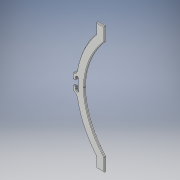
# Autodesk Inventor part: Baseplate_aussen
Saved by Autodesk Inventor 2018 (Build 220112000, 112)
## iProperties
Created: 2020-01-15
Part Number: Baseplate_aussen
Material: Generisch
Document SubType Name: Modeling
Designer: maxse
Density: 1 g/cm^3
Appearance: Vorgabe
Author: maxse
Autodesk Inventor part; units mm, degrees
ref_plane "YZ Plane" through (0, 0, 0) normal (1, 0, 0) x (0, 1, 0)
ref_plane "XZ Plane" through (0, 0, 0) normal (0, 1, 0) x (-1, 0, 0)
ref_plane "XY Plane" through (0, 0, 0) normal (0, 0, 1) x (1, 0, 0)
sketch "Skizze1" plane through (0, 0, 0) normal (0, 1, 0) x (-1, 0, 0)
  arc A0 (39, 0) -> (0, 95) centre (-110.879, -6.024) ccw
  line L0 (0, 95) -> (0, 120)
  line L1 (0, 120) -> (15, 120)
  line L2 (15, 120) -> (15, 100.6336)
  arc A1 (54, 0) -> (15, 100.6336) centre (-110.879, -6.024) ccw
  line L3 (39, 0) -> (54, 0)
  line L4 (0, 0) -> (39, 0)
  line L5 (59, 0) -> (59, 15)
  line L6 (59, 15) -> (52.765, 15)
  line L7 (59, 0) -> (54, 0)
  dimension "d0" = 25
  dimension "d2" = 15
  dimension "d4" = 54
  dimension "d5" = 0
  dimension "d6" = 120
  dimension "d7" = 150
  dimension "d9" = 5
  dimension "d10" = 15
  dimension "d11" = 15
  constraints: 16 end point, 6 point on circle, 3 perpendicular, 2 centre point, 2 horizontal, 2 vertical, 1 collinear, 1 concentric
  measures "d0" distance of L0.start L0.end
  measures "d2" distance of L0.end L1.end
  measures "d4" distance of L3.end L4.start
  measures "d5" distance from line of L4.start L0
  measures "d6" distance from line of L4.start L1
  measures "d7" radius of A0
  measures "d9" distance of L3.end L5.start
  measures "d10" distance of L3.end L3.start
  measures "d11" distance of L5.start L5.end
extrude "Extrusion1" add sketch "Skizze1" along normal blind 4
mirror "Spiegeln1" about plane through (-54, 0, 0) normal (0, 0, -1) of "Extrusion1"
sketch "Skizze2" plane through (0, 0, 0) normal (0, -1, 0) x (1, 0, 0)
  line L0 (-59, 15) -> (-59, -15) projected
  line L1 (-59, -5) -> (-54, -5)
  line L2 (-54, -5) -> (-54, -9.5)
  line L3 (-59, 5) -> (-54, 5)
  line L4 (-54, 5) -> (-54, 9.5)
  line L5 (-49, -9.5) -> (-49, 9.5)
  arc A0 (-49, 9.5) -> (-54, 9.5) centre (-51.5, 9.5) ccw
  arc A1 (-54, -9.5) -> (-49, -9.5) centre (-51.5, -9.5) ccw
  point P0 (0, 0)
  dimension "d15" = 10
  dimension "d16" = 5
  dimension "d17" = 10
  dimension "d18" = 5
  dimension "d19" = 5
  dimension "d20" = 24
  dimension "d21" = 4.5
  constraints: 10 end point, 4 point on circle, 4 tangent, 2 centre point, 2 horizontal, 2 point on line, 2 vertical, 1 perpendicular
  measures "d15" distance between parallel lines of L5 L0
  measures "d16" distance between parallel lines of L5 L2
  measures "d17" distance between parallel lines of L3 L1
  measures "d18" distance of L3.start L3.end
  measures "d19" distance from line of point (0, 0) L3
  measures "d21" distance from line of L1 A1.centre
extrude "Extrusion2" cut sketch "Skizze2" against normal blind 4
fillet "Rundung1" radius 10 3 edges at (-52.765, 2, -15) (-52.765, 2, 15) (-39, 2, 0)
fillet "Rundung2" radius 1 46 edges at (-7.5, 4, -120) (0, 4, -107.5) (-15, 4, -110.3168) (-7.5, 0, -120) (0, 0, -107.5) (-15, 0, -110.3168) (-54.0935, 4, -17.8718) (-38.4134, 4, -64.2123) (-54.0935, 0, -17.8718) (-38.4134, 0, -64.2123) (-38.9913, 4, 0) (-27.8012, 4, 51.1406) (-27.8012, 4, -51.1406) (-38.9913, 0, 0) (-27.8012, 0, 51.1406) (-27.8012, 0, -51.1406) (-54.0935, 4, 17.8718) (-38.4134, 4, 64.2123) (-54.0935, 0, 17.8718) (-38.4134, 0, 64.2123) (-59, 4, 10) (-59, 0, 10) (-59, 0, -10) (-59, 4, -10) (-59, 2, -5) (-59, 2, 5) (-54, 2, 5) (-54, 2, -5) (-56.5, 4, -5) (-56.5, 4, 5) (-51.5, 4, 12) (-54, 4, 7.25) (-51.5, 4, -12) (-54, 4, -7.25) (-49, 4, 0) (-51.5, 0, -12) (-54, 0, -7.25) (-51.5, 0, 12) (-54, 0, 7.25) (-49, 0, 0) (-15, 4, 110.3168) (-15, 0, 110.3168) (-7.5, 4, 120) (-7.5, 0, 120) (0, 0, 107.5) (0, 4, 107.5)
sketch "Skizze3" plane through (0, 4, 0) normal (0, 1, 0) x (1, 0, 0)
  line L0 (-45.0909, 10.6088) -> (-45.0909, 11.0512)
  line L1 (-45.0909, 11.0512) -> (-44.8243, 11.0512)
  spline S0 degree 2 poles (-44.8243, 11.0512) (-44.9094, 11.1533) (-45.0228, 11.3036) (-45.0711, 11.4058) knots 0 0 0 1 2 2 2
  spline S1 degree 2 poles (-45.0711, 11.4058) (-45.1164, 11.4994) (-45.1647, 11.7007) (-45.1647, 11.834) knots 0 0 0 1 2 2 2
  spline S2 degree 2 poles (-45.1647, 11.834) (-45.1647, 12.0496) (-44.986, 12.4126) (-44.813, 12.5403) knots 0 0 0 1 2 2 2
  spline S3 degree 2 poles (-44.813, 12.5403) (-44.6399, 12.6679) (-44.1294, 12.8097) (-43.7976, 12.8097) knots 0 0 0 1 2 2 2
  spline S4 degree 2 poles (-43.7976, 12.8097) (-43.4515, 12.8097) (-42.9467, 12.631) (-42.7566, 12.475) knots 0 0 0 1 2 2 2
  spline S5 degree 2 poles (-42.7566, 12.475) (-42.5865, 12.3304) (-42.3908, 11.9248) (-42.3908, 11.7007) knots 0 0 0 1 2 2 2
  spline S6 degree 2 poles (-42.3908, 11.7007) (-42.3908, 11.505) (-42.4787, 11.2129) (-42.5694, 11.0512) knots 0 0 0 1 2 2 2
  line L2 (-42.5694, 11.0512) -> (-41.4349, 11.0512)
  line L3 (-41.4349, 11.0512) -> (-41.4349, 10.6088)
  line L4 (-41.4349, 10.6088) -> (-45.0909, 10.6088)
  line L5 (-44.4528, 11.0512) -> (-42.9353, 11.0512)
  spline S7 degree 2 poles (-42.9353, 11.0512) (-42.8559, 11.2157) (-42.7964, 11.4767) (-42.7964, 11.627) knots 0 0 0 1 2 2 2
  spline S8 degree 2 poles (-42.7964, 11.627) (-42.7964, 11.9673) (-43.3069, 12.3531) (-43.7891, 12.3531) knots 0 0 0 1 2 2 2
  spline S9 degree 2 poles (-43.7891, 12.3531) (-44.2542, 12.3531) (-44.7449, 12.0581) (-44.7449, 11.7319) knots 0 0 0 1 2 2 2
  spline S10 degree 2 poles (-44.7449, 11.7319) (-44.7449, 11.5589) (-44.5861, 11.2072) (-44.4528, 11.0512) knots 0 0 0 1 2 2 2
  spline S11 degree 2 poles (-45.1505, 8.8276) (-45.1505, 9.4572) (-44.4442, 10.1493) (-43.7919, 10.1493) knots 0 0 0 1 2 2 2
  spline S12 degree 2 poles (-43.7919, 10.1493) (-43.1509, 10.1493) (-42.3908, 9.4771) (-42.3908, 8.9353) knots 0 0 0 1 2 2 2
  spline S13 degree 2 poles (-42.3908, 8.9353) (-42.3908, 8.6914) (-42.5326, 8.3142) (-42.6829, 8.1752) knots 0 0 0 1 2 2 2
  spline S14 degree 2 poles (-42.6829, 8.1752) (-42.8332, 8.0334) (-43.2672, 7.8831) (-43.582, 7.8831) knots 0 0 0 1 2 2 2
  line L6 (-43.582, 7.8831) -> (-43.8231, 7.8831)
  line L7 (-43.8231, 7.8831) -> (-43.8231, 9.7011)
  spline S15 degree 2 poles (-43.8231, 9.7011) (-44.2797, 9.7011) (-44.7647, 9.2417) (-44.7647, 8.8332) knots 0 0 0 1 2 2 2
  spline S16 degree 2 poles (-44.7647, 8.8332) (-44.7647, 8.6886) (-44.6995, 8.4078) (-44.6485, 8.2943) knots 0 0 0 1 2 2 2
  spline S17 degree 2 poles (-44.6485, 8.2943) (-44.5917, 8.1752) (-44.4925, 8.0107) (-44.4471, 7.9568) knots 0 0 0 1 2 2 2
  line L8 (-44.4471, 7.9568) -> (-44.4471, 7.9313)
  line L9 (-44.4471, 7.9313) -> (-44.9293, 7.9313)
  spline S18 degree 2 poles (-44.9293, 7.9313) (-44.9605, 8.0079) (-45.0512, 8.2404) (-45.0767, 8.3312) knots 0 0 0 1 2 2 2
  spline S19 degree 2 poles (-45.0767, 8.3312) (-45.1136, 8.4588) (-45.1505, 8.6687) (-45.1505, 8.8276) knots 0 0 0 1 2 2 2
  spline S20 degree 2 poles (-43.4856, 8.3142) (-43.3069, 8.3199) (-43.0459, 8.3936) (-42.958, 8.4645) knots 0 0 0 1 2 2 2
  spline S21 degree 2 poles (-42.958, 8.4645) (-42.8587, 8.5411) (-42.7538, 8.7822) (-42.7538, 8.9609) knots 0 0 0 1 2 2 2
  spline S22 degree 2 poles (-42.7538, 8.9609) (-42.7538, 9.1367) (-42.8587, 9.3835) (-42.9609, 9.4856) knots 0 0 0 1 2 2 2
  spline S23 degree 2 poles (-42.9609, 9.4856) (-43.0658, 9.5848) (-43.3182, 9.687) (-43.4856, 9.7011) knots 0 0 0 1 2 2 2
  line L10 (-43.4856, 9.7011) -> (-43.4856, 8.3142)
  spline S24 degree 2 poles (-45.1533, 6.7259) (-45.1533, 6.9896) (-45.0115, 7.4463) (-44.9321, 7.5966) knots 0 0 0 1 2 2 2
  line L11 (-44.9321, 7.5966) -> (-44.4357, 7.5966)
  line L12 (-44.4357, 7.5966) -> (-44.4357, 7.5739)
  spline S25 degree 2 poles (-44.4357, 7.5739) (-44.4811, 7.5172) (-44.5889, 7.364) (-44.6485, 7.2364) knots 0 0 0 1 2 2 2
  spline S26 degree 2 poles (-44.6485, 7.2364) (-44.7023, 7.1258) (-44.7818, 6.8535) (-44.7818, 6.7088) knots 0 0 0 1 2 2 2
  spline S27 degree 2 poles (-44.7818, 6.7088) (-44.7818, 6.6039) (-44.7335, 6.3628) (-44.6938, 6.3061) knots 0 0 0 1 2 2 2
  spline S28 degree 2 poles (-44.6938, 6.3061) (-44.6399, 6.2238) (-44.518, 6.1501) (-44.3932, 6.1501) knots 0 0 0 1 2 2 2
  spline S29 degree 2 poles (-44.3932, 6.1501) (-44.2372, 6.1501) (-44.0755, 6.3203) (-44.0216, 6.5387) knots 0 0 0 1 2 2 2
  spline S30 degree 2 poles (-44.0216, 6.5387) (-44.0018, 6.6237) (-43.9451, 6.896) (-43.9139, 7.0123) knots 0 0 0 1 2 2 2
  spline S31 degree 2 poles (-43.9139, 7.0123) (-43.8259, 7.313) (-43.4629, 7.5853) (-43.2048, 7.5853) knots 0 0 0 1 2 2 2
  spline S32 degree 2 poles (-43.2048, 7.5853) (-42.8474, 7.5853) (-42.4021, 7.0492) (-42.4021, 6.6067) knots 0 0 0 1 2 2 2
  spline S33 degree 2 poles (-42.4021, 6.6067) (-42.4021, 6.3883) (-42.5099, 5.9459) (-42.5921, 5.7955) knots 0 0 0 1 2 2 2
  line L13 (-42.5921, 5.7955) -> (-43.0658, 5.7955)
  line L14 (-43.0658, 5.7955) -> (-43.0658, 5.8182)
  spline S34 degree 2 poles (-43.0658, 5.8182) (-42.9297, 5.9884) (-42.7737, 6.4025) (-42.7737, 6.6152) knots 0 0 0 1 2 2 2
  spline S35 degree 2 poles (-42.7737, 6.6152) (-42.7737, 6.8336) (-42.958, 7.1343) (-43.1424, 7.1343) knots 0 0 0 1 2 2 2
  spline S36 degree 2 poles (-43.1424, 7.1343) (-43.3097, 7.1343) (-43.4714, 6.9556) (-43.5224, 6.7571) knots 0 0 0 1 2 2 2
  spline S37 degree 2 poles (-43.5224, 6.7571) (-43.548, 6.6606) (-43.599, 6.4167) (-43.6302, 6.2834) knots 0 0 0 1 2 2 2
  spline S38 degree 2 poles (-43.6302, 6.2834) (-43.704, 5.9941) (-44.0415, 5.6991) (-44.3336, 5.6991) knots 0 0 0 1 2 2 2
  spline S39 degree 2 poles (-44.3336, 5.6991) (-44.5038, 5.6991) (-44.8045, 5.8324) (-44.9151, 5.9629) knots 0 0 0 1 2 2 2
  spline S40 degree 2 poles (-44.9151, 5.9629) (-45.0314, 6.1019) (-45.1533, 6.4564) (-45.1533, 6.7259) knots 0 0 0 1 2 2 2
  line L15 (-45.0909, 4.8369) -> (-45.0909, 5.2793)
  line L16 (-45.0909, 5.2793) -> (-42.4645, 5.2793)
  line L17 (-42.4645, 5.2793) -> (-42.4645, 4.8369)
  line L18 (-42.4645, 4.8369) -> (-45.0909, 4.8369)
  line L19 (-42.0277, 4.8057) -> (-42.0277, 5.3077)
  line L20 (-42.0277, 5.3077) -> (-41.5682, 5.3077)
  line L21 (-41.5682, 5.3077) -> (-41.5682, 4.8057)
  line L22 (-41.5682, 4.8057) -> (-42.0277, 4.8057)
  spline S41 degree 2 poles (-45.5107, 4.0938) (-45.5305, 4.0484) (-45.5929, 3.8754) (-45.6185, 3.7648) knots 0 0 0 1 2 2 2
  spline S42 degree 2 poles (-45.6185, 3.7648) (-45.6497, 3.6428) (-45.6865, 3.4357) (-45.6865, 3.3138) knots 0 0 0 1 2 2 2
  spline S43 degree 2 poles (-45.6865, 3.3138) (-45.6865, 3.1096) (-45.5788, 2.8259) (-45.4823, 2.7465) knots 0 0 0 1 2 2 2
  spline S44 degree 2 poles (-45.4823, 2.7465) (-45.3859, 2.6699) (-45.1335, 2.6104) (-44.9718, 2.6104) knots 0 0 0 1 2 2 2
  line L23 (-44.9718, 2.6104) -> (-44.7421, 2.6104)
  spline S45 degree 2 poles (-44.7421, 2.6104) (-44.8981, 2.7891) (-45.0455, 3.1323) (-45.0455, 3.3904) knots 0 0 0 1 2 2 2
  spline S46 degree 2 poles (-45.0455, 3.3904) (-45.0455, 3.8385) (-44.379, 4.3689) (-43.7522, 4.3689) knots 0 0 0 1 2 2 2
  spline S47 degree 2 poles (-43.7522, 4.3689) (-43.426, 4.3689) (-42.9211, 4.1845) (-42.7425, 4.0314) knots 0 0 0 1 2 2 2
  spline S48 degree 2 poles (-42.7425, 4.0314) (-42.5751, 3.8839) (-42.3908, 3.4783) (-42.3908, 3.2627) knots 0 0 0 1 2 2 2
  spline S49 degree 2 poles (-42.3908, 3.2627) (-42.3908, 3.0585) (-42.4872, 2.7607) (-42.5751, 2.6104) knots 0 0 0 1 2 2 2
  line L24 (-42.5751, 2.6104) -> (-42.4645, 2.5848)
  line L25 (-42.4645, 2.5848) -> (-42.4645, 2.1679)
  line L26 (-42.4645, 2.1679) -> (-44.7903, 2.1679)
  spline S50 degree 2 poles (-44.7903, 2.1679) (-45.4596, 2.1679) (-46.0836, 2.7494) (-46.0836, 3.3478) knots 0 0 0 1 2 2 2
  spline S51 degree 2 poles (-46.0836, 3.3478) (-46.0836, 3.5407) (-46.0212, 3.9434) (-45.9702, 4.1165) knots 0 0 0 1 2 2 2
  line L27 (-45.9702, 4.1165) -> (-45.5107, 4.1165)
  line L28 (-45.5107, 4.1165) -> (-45.5107, 4.0938)
  line L29 (-44.379, 2.6104) -> (-42.9353, 2.6104)
  spline S52 degree 2 poles (-42.9353, 2.6104) (-42.8559, 2.7749) (-42.7878, 3.0528) (-42.7878, 3.1918) knots 0 0 0 1 2 2 2
  spline S53 degree 2 poles (-42.7878, 3.1918) (-42.7878, 3.5265) (-43.2814, 3.9122) (-43.7437, 3.9122) knots 0 0 0 1 2 2 2
  spline S54 degree 2 poles (-43.7437, 3.9122) (-44.1805, 3.9122) (-44.6371, 3.6201) (-44.6371, 3.2911) knots 0 0 0 1 2 2 2
  spline S55 degree 2 poles (-44.6371, 3.2911) (-44.6371, 3.1181) (-44.501, 2.755) (-44.379, 2.6104) knots 0 0 0 1 2 2 2
  line L30 (-45.0909, -0.5351) -> (-45.0909, -0.0926)
  line L31 (-45.0909, -0.0926) -> (-43.5934, -0.0926)
  spline S56 degree 2 poles (-43.5934, -0.0926) (-43.4118, -0.0926) (-43.0998, -0.0586) (-43.0062, -0.0075) knots 0 0 0 1 2 2 2
  spline S57 degree 2 poles (-43.0062, -0.0075) (-42.907, 0.0464) (-42.8105, 0.2392) (-42.8105, 0.4037) knots 0 0 0 1 2 2 2
  spline S58 degree 2 poles (-42.8105, 0.4037) (-42.8105, 0.5682) (-42.9864, 0.9171) (-43.1282, 1.0844) knots 0 0 0 1 2 2 2
  line L32 (-43.1282, 1.0844) -> (-45.0909, 1.0844)
  line L33 (-45.0909, 1.0844) -> (-45.0909, 1.5269)
  line L34 (-45.0909, 1.5269) -> (-42.4645, 1.5269)
  line L35 (-42.4645, 1.5269) -> (-42.4645, 1.0844)
  line L36 (-42.4645, 1.0844) -> (-42.7566, 1.0844)
  spline S59 degree 2 poles (-42.7566, 1.0844) (-42.578, 0.8859) (-42.3908, 0.503) (-42.3908, 0.2874) knots 0 0 0 1 2 2 2
  spline S60 degree 2 poles (-42.3908, 0.2874) (-42.3908, -0.0983) (-42.9013, -0.5351) (-43.3863, -0.5351) knots 0 0 0 1 2 2 2
  line L37 (-43.3863, -0.5351) -> (-45.0909, -0.5351)
  spline S61 degree 2 poles (-45.1505, -2.2964) (-45.1505, -1.6668) (-44.4442, -0.9747) (-43.7919, -0.9747) knots 0 0 0 1 2 2 2
  spline S62 degree 2 poles (-43.7919, -0.9747) (-43.1509, -0.9747) (-42.3908, -1.6469) (-42.3908, -2.1887) knots 0 0 0 1 2 2 2
  spline S63 degree 2 poles (-42.3908, -2.1887) (-42.3908, -2.4326) (-42.5326, -2.8098) (-42.6829, -2.9488) knots 0 0 0 1 2 2 2
  spline S64 degree 2 poles (-42.6829, -2.9488) (-42.8332, -3.0906) (-43.2672, -3.2409) (-43.582, -3.2409) knots 0 0 0 1 2 2 2
  line L38 (-43.582, -3.2409) -> (-43.8231, -3.2409)
  line L39 (-43.8231, -3.2409) -> (-43.8231, -1.4229)
  spline S65 degree 2 poles (-43.8231, -1.4229) (-44.2797, -1.4229) (-44.7647, -1.8823) (-44.7647, -2.2908) knots 0 0 0 1 2 2 2
  spline S66 degree 2 poles (-44.7647, -2.2908) (-44.7647, -2.4354) (-44.6995, -2.7162) (-44.6485, -2.8297) knots 0 0 0 1 2 2 2
  spline S67 degree 2 poles (-44.6485, -2.8297) (-44.5917, -2.9488) (-44.4925, -3.1133) (-44.4471, -3.1672) knots 0 0 0 1 2 2 2
  line L40 (-44.4471, -3.1672) -> (-44.4471, -3.1927)
  line L41 (-44.4471, -3.1927) -> (-44.9293, -3.1927)
  spline S68 degree 2 poles (-44.9293, -3.1927) (-44.9605, -3.1161) (-45.0512, -2.8835) (-45.0767, -2.7928) knots 0 0 0 1 2 2 2
  spline S69 degree 2 poles (-45.0767, -2.7928) (-45.1136, -2.6652) (-45.1505, -2.4553) (-45.1505, -2.2964) knots 0 0 0 1 2 2 2
  spline S70 degree 2 poles (-43.4856, -2.8098) (-43.3069, -2.8041) (-43.0459, -2.7304) (-42.958, -2.6595) knots 0 0 0 1 2 2 2
  spline S71 degree 2 poles (-42.958, -2.6595) (-42.8587, -2.5829) (-42.7538, -2.3418) (-42.7538, -2.1631) knots 0 0 0 1 2 2 2
  spline S72 degree 2 poles (-42.7538, -2.1631) (-42.7538, -1.9873) (-42.8587, -1.7405) (-42.9609, -1.6384) knots 0 0 0 1 2 2 2
  spline S73 degree 2 poles (-42.9609, -1.6384) (-43.0658, -1.5391) (-43.3182, -1.437) (-43.4856, -1.4229) knots 0 0 0 1 2 2 2
  line L42 (-43.4856, -1.4229) -> (-43.4856, -2.8098)
  line L43 (-45.0909, -5.7085) -> (-45.0909, -5.266)
  line L44 (-45.0909, -5.266) -> (-44.8243, -5.266)
  spline S74 degree 2 poles (-44.8243, -5.266) (-44.9094, -5.1639) (-45.0228, -5.0136) (-45.0711, -4.9115) knots 0 0 0 1 2 2 2
  spline S75 degree 2 poles (-45.0711, -4.9115) (-45.1164, -4.8179) (-45.1647, -4.6165) (-45.1647, -4.4832) knots 0 0 0 1 2 2 2
  spline S76 degree 2 poles (-45.1647, -4.4832) (-45.1647, -4.2677) (-44.986, -3.9046) (-44.813, -3.777) knots 0 0 0 1 2 2 2
  spline S77 degree 2 poles (-44.813, -3.777) (-44.6399, -3.6494) (-44.1294, -3.5075) (-43.7976, -3.5075) knots 0 0 0 1 2 2 2
  spline S78 degree 2 poles (-43.7976, -3.5075) (-43.4515, -3.5075) (-42.9467, -3.6862) (-42.7566, -3.8422) knots 0 0 0 1 2 2 2
  spline S79 degree 2 poles (-42.7566, -3.8422) (-42.5865, -3.9869) (-42.3908, -4.3925) (-42.3908, -4.6165) knots 0 0 0 1 2 2 2
  spline S80 degree 2 poles (-42.3908, -4.6165) (-42.3908, -4.8122) (-42.4787, -5.1044) (-42.5694, -5.266) knots 0 0 0 1 2 2 2
  line L45 (-42.5694, -5.266) -> (-41.4349, -5.266)
  line L46 (-41.4349, -5.266) -> (-41.4349, -5.7085)
  line L47 (-41.4349, -5.7085) -> (-45.0909, -5.7085)
  line L48 (-44.4528, -5.266) -> (-42.9353, -5.266)
  spline S81 degree 2 poles (-42.9353, -5.266) (-42.8559, -5.1015) (-42.7964, -4.8406) (-42.7964, -4.6903) knots 0 0 0 1 2 2 2
  spline S82 degree 2 poles (-42.7964, -4.6903) (-42.7964, -4.3499) (-43.3069, -3.9642) (-43.7891, -3.9642) knots 0 0 0 1 2 2 2
  spline S83 degree 2 poles (-43.7891, -3.9642) (-44.2542, -3.9642) (-44.7449, -4.2592) (-44.7449, -4.5853) knots 0 0 0 1 2 2 2
  spline S84 degree 2 poles (-44.7449, -4.5853) (-44.7449, -4.7583) (-44.5861, -5.11) (-44.4528, -5.266) knots 0 0 0 1 2 2 2
  spline S85 degree 2 poles (-43.7352, -10.0537) (-44.379, -10.0537) (-45.1647, -9.4297) (-45.1647, -8.9589) knots 0 0 0 1 2 2 2
  spline S86 degree 2 poles (-45.1647, -8.9589) (-45.1647, -8.7462) (-45.0597, -8.4427) (-44.969, -8.2952) knots 0 0 0 1 2 2 2
  line L49 (-44.969, -8.2952) -> (-45.0909, -8.2669)
  line L50 (-45.0909, -8.2669) -> (-45.0909, -7.8528)
  line L51 (-45.0909, -7.8528) -> (-41.4349, -7.8528)
  line L52 (-41.4349, -7.8528) -> (-41.4349, -8.2952)
  line L53 (-41.4349, -8.2952) -> (-42.7396, -8.2952)
  spline S87 degree 2 poles (-42.7396, -8.2952) (-42.5893, -8.4626) (-42.3908, -8.8511) (-42.3908, -9.0979) knots 0 0 0 1 2 2 2
  spline S88 degree 2 poles (-42.3908, -9.0979) (-42.3908, -9.5432) (-43.1027, -10.0537) (-43.7352, -10.0537) knots 0 0 0 1 2 2 2
  spline S89 degree 2 poles (-43.7692, -9.5971) (-43.2984, -9.5971) (-42.8105, -9.3106) (-42.8105, -8.9929) knots 0 0 0 1 2 2 2
  spline S90 degree 2 poles (-42.8105, -8.9929) (-42.8105, -8.8143) (-42.9807, -8.4455) (-43.1112, -8.2952) knots 0 0 0 1 2 2 2
  line L54 (-43.1112, -8.2952) -> (-44.6173, -8.2952)
  spline S91 degree 2 poles (-44.6173, -8.2952) (-44.6995, -8.4626) (-44.7676, -8.7207) (-44.7676, -8.8738) knots 0 0 0 1 2 2 2
  spline S92 degree 2 poles (-44.7676, -8.8738) (-44.7676, -9.2113) (-44.2882, -9.5971) (-43.7692, -9.5971) knots 0 0 0 1 2 2 2
  line L55 (-42.4645, -12.5752) -> (-46.0581, -11.1627)
  line L56 (-46.0581, -11.1627) -> (-46.0581, -10.6891)
  line L57 (-46.0581, -10.6891) -> (-44.9633, -11.1599)
  line L58 (-44.9633, -11.1599) -> (-42.4645, -10.2069)
  line L59 (-42.4645, -10.2069) -> (-42.4645, -10.6834)
  line L60 (-42.4645, -10.6834) -> (-44.4102, -11.401)
  line L61 (-44.4102, -11.401) -> (-42.4645, -12.1157)
  line L62 (-42.4645, -12.1157) -> (-42.4645, -12.5752)
  point P0 (0, 0)
  point P1 (-41.4349, 12.9487)
  constraints: 1 other
extrude "Extrusion3" add sketch "Skizze3" along normal blind 1
